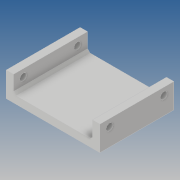
# Autodesk Inventor part: base_cloison
Saved by Autodesk Inventor 2019 (Build 230136000, 136)
## iProperties
Created: 2020-07-07
Part Number: base_cloison
Material: Générique
Document SubType Name: Modeling
Designer: Theo
Density: 1 g/cm^3
Appearance: Par défaut
Author: Theo
Autodesk Inventor part; units mm, degrees
ref_plane "YZ Plane" through (0, 0, 0) normal (1, 0, 0) x (0, 1, 0)
ref_plane "XZ Plane" through (0, 0, 0) normal (0, 1, 0) x (-1, 0, 0)
ref_plane "XY Plane" through (0, 0, 0) normal (0, 0, 1) x (1, 0, 0)
sketch "Esquisse1" plane through (0, 0, 0) normal (0, 1, 0) x (-1, 0, 0)
  line L0 (38, 30) -> (-38, 30)
  line L1 (-38, 30) -> (-38, -30)
  line L2 (-38, -30) -> (38, -30)
  line L3 (38, -30) -> (38, 30)
  line L4 (38, 30) -> (-38, -30) construction
  line L5 (-38, 30) -> (38, -30) construction
  point P0 (0, 0)
  dimension "d0" = 76
  dimension "d1" = 60
  constraints: 12 end point, 2 midpoint, 2 parallel, 1 horizontal, 1 perpendicular
  measures "d0" distance of L1.end L2.end
  measures "d1" distance of L0.end L1.end
extrude "Extrusion1" add sketch "Esquisse1" along normal blind 6
sketch "Esquisse2" plane through (0, 6, 0) normal (0, 1, 0) x (1, 0, 0)
  line L0 (38, 30) -> (-38, 30) projected
  line L1 (-38, -30) -> (38, -30) projected
  line L2 (-38, 30) -> (-32, 30)
  line L3 (-32, 30) -> (-32, -30)
  line L4 (-32, -30) -> (-38, -30)
  line L5 (-38, -30) -> (-38, 30)
  line L6 (38, 30) -> (32, 30)
  line L7 (32, 30) -> (32, -30)
  line L8 (32, -30) -> (38, -30)
  line L9 (38, -30) -> (38, 30)
  point P0 (0, 0)
  dimension "d4" = 6
  dimension "d5" = 6
  constraints: 16 end point, 4 parallel, 2 horizontal, 2 perpendicular, 2 point on line
  measures "d4" distance of L0.end L2.end
  measures "d5" distance of L0.start L6.end
extrude "Extrusion2" add sketch "Esquisse2" along normal blind 14 contours L9 L1 L7 L0 | L3 L1 L5 L0
chamfer "Chanfrein1" distance 2 angle 45 2 edges at (-32, 6, 0) (32, 6, 0)
sketch "Esquisse4" plane through (38, 0, 30) normal (1, 0, 0) x (0, 0, -1)
  line L0 (0, 20) -> (60, 20) projected
  line L1 (60, 0) -> (60, 20) projected
  line L2 (0, 0) -> (0, 20) projected
  line L3 (0, 0) -> (60, 0) projected
  point P0 (30, 0)
  point P1 (52, 14)
  point P2 (8, 14)
  dimension "d11" = 6
  dimension "d12" = 8
  dimension "d13" = 8
  dimension "d21" = 14
  constraints: 1 horizontal alignment
  measures "d11" distance from line of L0 point (52, 14)
  measures "d12" distance from line of L1 point (52, 14)
  measures "d13" distance from line of point (8, 14) L2
  measures "d21" distance from line of L3 point (52, 14)
hole "Perçage1" at (38, 14, -22) at (38, 14, 22) direction (-1, 0, 0) diameter 5.5 end through all clearance for "Vis d'assemblage à tête hexagonale ISO 24017" size "M5" standard "ISO"
equation "\"d13\" = d12"
